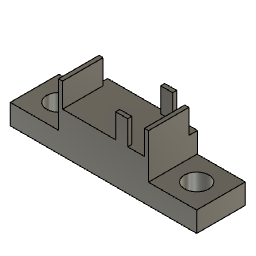
LimitBox (Autodesk Fusion 360 design; units mm, degrees)
Autodesk Fusion 360 part; units mm, degrees
note: some values were not read from the file. Chosen so that the rebuilt part matches the saved one: which bodies a step acts on. Set by a fixed rule: which sketch regions a step uses.
sketch "Sketch1" plane through (0, 0, 0) normal (0, 0, 1) x (1, 0, 0)
  line L0 (0, 0) -> (20, 0) construction
  line L1 (20, 10) -> (0, 10) construction
  circle A0 centre (5.5, 2.6799) radius 1 construction
  circle A1 centre (14.5, 2.6799) radius 1 construction
  line L2 (10, 10) -> (10, -5.8296) construction
  line L3 (20, 10) -> (20, 0) construction
  line L4 (0, 0) -> (0, 10) construction
  line L5 (20.1, 10) -> (21.1, 10)
  line L6 (21.1, 10) -> (21.1, 0)
  line L7 (21.1, 0) -> (20.1, 0)
  line L8 (20.1, 0) -> (20.1, 10)
  line L9 (0, 10) -> (0, 0) construction
  line L10 (-1.1, 0) -> (-0.1, 0)
  line L11 (-0.1, 10) -> (-1.1, 10)
  line L12 (-1.1, 10) -> (-1.1, 0)
  line L13 (-0.1, 0) -> (-0.1, 10)
  line L14 (13, 12.1) -> (16, 12.1)
  line L15 (16, 12.1) -> (16, 11.1)
  line L16 (16, 11.1) -> (13, 11.1)
  line L17 (13, 11.1) -> (13, 12.1)
  line L18 (13, 1) -> (16, 1)
  line L19 (16, 1) -> (16, 0)
  line L20 (16, 0) -> (13, 0)
  line L21 (13, 0) -> (13, 1)
  line L22 (14.5, 12.1) -> (14.5, 11.1) construction
  line L23 (14.5, 1) -> (14.5, 0) construction
  dimension "d1" = 10
  dimension "d2" = 20
  dimension "d3" = 2
  dimension "d4" = 9
  dimension "d32" = 0.1
  dimension "d33" = 1
  dimension "d34" = 1.1
  dimension "d35" = 10.1
  dimension "d36" = 1
  dimension "d37" = 1
  dimension "d38" = 3
  dimension "d39" = 3
  constraint horizontal L0
  constraint horizontal L1
  constraint coincident L0.start L4.start
  constraint equal A0 A1
  constraint midpoint L1 L2.start
  constraint perpendicular L1 L2
  constraint symmetric A0 A1 L2
  constraint perpendicular L0 L3
  constraint perpendicular L1 L4
  constraint horizontal L5
  constraint vertical L6
  constraint horizontal L7
  constraint vertical L8
  constraint collinear L1 L5
  constraint collinear L0 L7
  constraint symmetric L0.end L2 L0.start
  constraint symmetric L1.start L2 L1.end
  constraint symmetric L2 L5.start L11.start
  constraint symmetric L2 L5.end L11.end
  constraint symmetric L2 L6.end L10.start
  constraint symmetric L2 L7.end L10.end
  constraint horizontal L14
  constraint vertical L15
  constraint horizontal L16
  constraint vertical L17
  constraint horizontal L18
  constraint vertical L19
  constraint horizontal L20
  constraint vertical L21
  constraint midpoint L14 L22.start
  constraint midpoint L16 L22.end
  constraint midpoint L18 L23.start
  constraint midpoint L20 L23.end
  constraint vertical A1.centre L22.end
  constraint vertical L22.end L23.start
  measures "d1" distance of L0.start L1.end
  measures "d2" distance of L0.start L0.end
  measures "d3" diameter of A0
  measures "d4" distance of A0.centre A1.centre
  measures "d32" distance of L3 L8
  measures "d33" distance of L5.start L5.end
  measures "d34" distance of L1 L16
  measures "d35" distance of L16 L18
  measures "d36" distance of L18.end L19.end
  measures "d37" distance of L14.end L15.end
  measures "d38" distance of L14.start L14.end
  measures "d39" distance of L19 L21
extrude "Extrude1" add sketch "Sketch1" along normal blind 6 makes body 1 at (15, 11.1, 2) makes body 2 at (15, 0, 2) makes body 3 at (21.1, 6.6667, 2) makes body 4 at (-1.1, 6.6667, 2)
sketch "Sketch2" plane through (0, 0, 0) normal (0, 0, -1) x (1, 0, 0)
  line L0 (-1.1, -12.1) -> (21.1, -12.1)
  line L1 (21.1, -12.1) -> (21.1, 0)
  line L2 (21.1, 0) -> (-1.1, 0)
  line L3 (-1.1, 0) -> (-1.1, -12.1)
  line L4 (16, -12.1) -> (13, -12.1)
  line L5 (21.1, 0) -> (21.1, -10)
  line L6 (13, 0) -> (16, 0)
  line L7 (-1.1, -10) -> (-1.1, 0)
  constraint horizontal L0
  constraint vertical L1
  constraint horizontal L2
  constraint vertical L3
  constraint collinear L0 L4
  constraint collinear L1 L5
  constraint collinear L2 L6
  constraint collinear L3 L7
extrude "Extrude2" add sketch "Sketch2" along normal blind 10 bodies 1 2 3 4
sketch "Sketch5" plane through (0, 0, -10) normal (0, 0, -1) x (1, 0, 0)
  line L0 (-1, 0) -> (-13, 0)
  line L1 (-13, 0) -> (-13, -12)
  line L2 (-13, -12) -> (-1, -12)
  line L3 (-1, -12) -> (-1, 0)
  circle A0 centre (-7, -6) radius 3
  line L4 (10, 0) -> (10, 4.7186) construction
  line L5 (33, -12) -> (21, -12)
  circle A1 centre (27, -6) radius 3
  line L6 (21, -12) -> (21, 0)
  line L7 (21, 0) -> (33, 0)
  line L8 (21, 0) -> (21, -12)
  line L9 (33, 0) -> (33, -12)
  line L10 (-1.1, -12.1) -> (21.1, -12.1)
  line L11 (21.1, -12.1) -> (21.1, 0)
  line L12 (21.1, 0) -> (-1.1, 0)
  line L13 (-1.1, 0) -> (-1.1, -12.1)
  point P0 (20, 0)
  dimension "d27" = 6
  dimension "d28" = 6
  dimension "d29" = 6
  constraint horizontal L0
  constraint vertical L1
  constraint horizontal L2
  constraint vertical L3
  constraint equal L0 L1
  constraint symmetric origin L4 P0
  constraint symmetric L0.start L4 L6.end
  constraint symmetric L0.end L4 L7.end
  constraint symmetric L1.end L4 L5.start
  constraint symmetric L2.end L4 L5.end
  constraint symmetric A0 L4 A1
  measures "d27" diameter of A0
  measures "d28" distance of L0 A0.centre
  measures "d29" distance of L1 A0.centre
extrude "Extrude5" add sketch "Sketch5" against normal blind 5 contours L0 L1 L2 L13 | L5 L7 L9 L11 bodies 1
